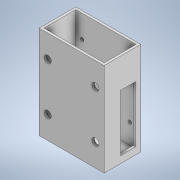
# Autodesk Inventor part: piCaseAttachesToTripodClamp
Saved by Autodesk Inventor 2021.2 (Build 252289000, 289)
## iProperties
Created: 2021-02-07
Part Number: piCaseAttachesToTripodClamp
Material: Generic
Document SubType Name: Modeling
Designer: robst
Density: 1 g/cm^3
Appearance: Default
Author: robst
Autodesk Inventor part; units mm, degrees
ref_plane "YZ Plane" through (0, 0, 0) normal (1, 0, 0) x (0, 1, 0)
ref_plane "XZ Plane" through (0, 0, 0) normal (0, 1, 0) x (-1, 0, 0)
ref_plane "XY Plane" through (0, 0, 0) normal (0, 0, 1) x (1, 0, 0)
sketch "Sketch14" plane through (0, 0, 0) normal (0, 0, 1) x (1, 0, 0)
  line L0 (-34.54, -49.54) -> (34.54, -49.54)
  line L1 (34.54, -49.54) -> (34.54, 49.54)
  line L2 (34.54, 49.54) -> (-34.54, 49.54)
  line L3 (-34.54, 49.54) -> (-34.54, -49.54)
  line L4 (-34.54, -49.54) -> (34.54, 49.54) construction
  line L5 (34.54, -49.54) -> (-34.54, 49.54) construction
  point P0 (0, 0)
  dimension "d66" = 69.08
  dimension "d67" = 99.08
  constraints: 12 end point, 2 midpoint, 2 parallel, 1 horizontal, 1 perpendicular
  measures "d66" distance of L0.start L0.end
  measures "d67" distance of L2.end L0.start
extrude "Extrusion9" add sketch "Sketch14" against normal blind 2.54
sketch "Sketch15" plane through (0, 0, 0) normal (0, 0, 1) x (1, 0, 0)
  line L0 (-34.54, -49.54) -> (-34.54, 49.54) projected
  line L1 (34.54, 49.54) -> (34.54, -49.54) projected
  line L2 (-34.54, -49.54) -> (34.54, -49.54)
  line L3 (34.54, -49.54) -> (34.54, 49.54)
  line L4 (34.54, 49.54) -> (-34.54, 49.54)
  line L5 (-34.54, 49.54) -> (-34.54, -49.54)
  line L6 (-32, -47) -> (32, -47)
  line L7 (32, -47) -> (32, 47)
  line L8 (32, 47) -> (-32, 47)
  line L9 (-32, 47) -> (-32, -47)
  line L10 (-32, -47) -> (32, 47) construction
  line L11 (32, -47) -> (-32, 47) construction
  point P0 (0, 0)
  point P1 (34.54, -49.54)
  dimension "d70" = 64
  dimension "d71" = 94
  constraints: 20 end point, 4 parallel, 2 horizontal, 2 midpoint, 2 perpendicular
  measures "d70" distance of L6.start L6.end
  measures "d71" distance of L8.end L6.start
extrude "Extrusion10" add sketch "Sketch15" along normal blind 34
sketch "Sketch16" plane through (0, 0, 34) normal (0, 0, 1) x (1, 0, 0)
  line L0 (-34.54, -49.54) -> (-34.54, 49.54) projected
  line L1 (34.54, 49.54) -> (34.54, -49.54) projected
  line L2 (-34.54, -49.54) -> (34.54, -49.54)
  line L3 (34.54, -49.54) -> (34.54, 49.54)
  line L4 (34.54, 49.54) -> (-34.54, 49.54)
  line L5 (-34.54, 49.54) -> (-34.54, -49.54)
  point P0 (0, 0)
  point P1 (34.54, -49.54)
  constraints: 8 end point, 2 parallel, 1 horizontal, 1 perpendicular
extrude "Extrusion11" add sketch "Sketch16" along normal blind 2.54
sketch "Sketch17" plane through (-34.54, 49.54, -2.54) normal (0, 1, 0) x (1, 0, 0)
  line L0 (66.54, -2.54) -> (66.54, -36.54) projected
  line L1 (2.54, -36.54) -> (66.54, -36.54) projected
  line L2 (2.54, -2.54) -> (2.54, -36.54) projected
  line L3 (66.54, -2.54) -> (2.54, -2.54) projected
  line L4 (2.54, -36.54) -> (66.54, -36.54)
  line L5 (66.54, -36.54) -> (66.54, -2.54)
  line L6 (66.54, -2.54) -> (2.54, -2.54)
  line L7 (2.54, -2.54) -> (2.54, -36.54)
  point P0 (34.54, -2.54)
  constraints: 8 end point, 2 parallel, 1 horizontal, 1 perpendicular
extrude "Extrusion12" cut sketch "Sketch17" against normal blind 2.54
sketch "Sketch18" plane through (34.54, -49.54, -2.54) normal (1, 0, 0) x (0, 0, -1)
  line L0 (-2.54, 2.54) -> (-2.54, 99.08) projected
  line L1 (-36.54, 99.08) -> (-36.54, 2.54) projected
  line L2 (-2.54, 2.54) -> (-36.54, 2.54) projected
  line L3 (-21.54, 7.54) -> (-5.54, 7.54)
  line L4 (-5.54, 7.54) -> (-5.54, 67.54)
  line L5 (-5.54, 67.54) -> (-21.54, 67.54)
  line L6 (-21.54, 67.54) -> (-21.54, 7.54)
  line L7 (-21.54, 7.54) -> (-5.54, 67.54) construction
  line L8 (-5.54, 7.54) -> (-21.54, 67.54) construction
  line L9 (-39.08, 0) -> (-39.08, 99.08) projected
  point P0 (-2.54, 49.54)
  point P1 (-13.54, 37.54)
  dimension "d78" = 5
  dimension "d79" = 3
  dimension "d80" = 15
  dimension "d81" = 65
  constraints: 12 end point, 2 midpoint, 2 parallel, 2 perpendicular
  measures "d78" distance between parallel lines of L3 L2
  measures "d79" distance between parallel lines of L4 L0
  measures "d80" distance between parallel lines of L6 L1
  measures "d81" distance between parallel lines of L5 L2
extrude "Extrusion13" cut sketch "Sketch18" against normal blind 2.54
sketch "Sketch19" plane through (0, 0, -2.54) normal (0, 0, -1) x (-1, 0, 0)
  line L0 (-25.4, -25.4) -> (25.4, -25.4) construction
  line L1 (25.4, -25.4) -> (25.4, 25.4) construction
  line L2 (25.4, 25.4) -> (-25.4, 25.4) construction
  line L3 (-25.4, 25.4) -> (-25.4, -25.4) construction
  line L4 (-25.4, -25.4) -> (25.4, 25.4) construction
  line L5 (25.4, -25.4) -> (-25.4, 25.4) construction
  point P0 (0, 0)
  dimension "d84" = 50.8
  dimension "d85" = 50.8
  constraints: 12 end point, 2 midpoint, 2 parallel, 1 horizontal, 1 perpendicular
  measures "d84" distance of L0.start L0.end
  measures "d85" distance of L2.end L0.start
hole "Hole3" at (25.4, 25.4, -2.54) at (-25.4, 25.4, -2.54) at (-25.4, -25.4, -2.54) at (25.4, -25.4, -2.54) direction (0, 0, 1) diameter 3.81 end through all clearance for "Flat Head Machine Screw (82)" size "#6" standard "Ansi Unified Screw Threads"
sketch "Sketch22" plane through (0, 0, 36.54) normal (0, 0, 1) x (1, 0, 0)
  circle A0 centre (-25.4, 25.4) radius 1.905 projected
  circle A1 centre (25.4, 25.4) radius 1.905 projected
  circle A2 centre (25.4, -25.4) radius 1.905 projected
  circle A3 centre (-25.4, -25.4) radius 1.905 projected
  point P0 (0, 0)
  constraints: 4 coincident
hole "Hole4" at (-25.4, 25.4, 36.54) at (25.4, 25.4, 36.54) at (25.4, -25.4, 36.54) at (-25.4, -25.4, 36.54) direction (0, 0, -1) diameter 7.62 depth 2.54
equation "\"d66\" = piBoxExteriorWidth"
equation "\"d67\" = piBoxExteriorLength"
equation "\"d68\" = piBoxWallThickness"
equation "\"d70\" = piBoxInteriorWidth"
equation "\"d71\" = piBoxInteriorLength"
equation "\"d72\" = piBoxInteriorHeight"
equation "\"d74\" = piBoxWallThickness"
equation "\"d76\" = piBoxWallThickness"
equation "\"d82\" = piBoxWallThickness"
equation "\"piBoxInteriorLength\" = 94"
equation "\"piBoxInteriorWidth\" = 64"
equation "\"piBoxInteriorHeight\" = 34"
equation "\"piBoxThickness\" = 3.175"
equation "\"piBoxWallThickness\" = 2.54"
equation "\"piBoxExteriorLength\" = piBoxInteriorLength + 2 * piBoxWallThickness"
equation "\"piBoxExteriorHeight\" = piBoxInteriorHeight + piBoxWallThickness"
equation "\"piBoxExteriorWidth\" = piBoxInteriorWidth + 2 * piBoxWallThickness"
body "Solid1"
body "Solid2"
